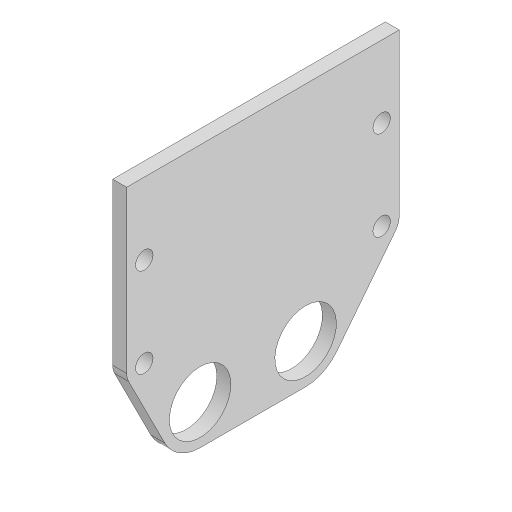
# Autodesk Inventor part: grabberPlate
Saved by Autodesk Inventor 2023 (Build 270158000, 158)
## iProperties
Created: 2022-09-10
Part Number: grabberPlate
Material: Generic
Document SubType Name: Modeling
Designer: deli
Density: 1 g/cm^3
Appearance: Default
Author: deli
Autodesk Inventor part; units mm, degrees
ref_plane "YZ Plane" through (0, 0, 0) normal (1, 0, 0) x (0, 1, 0)
ref_plane "XZ Plane" through (0, 0, 0) normal (0, 1, 0) x (-1, 0, 0)
ref_plane "XY Plane" through (0, 0, 0) normal (0, 0, 1) x (1, 0, 0)
sketch "Sketch1" plane through (0, 0, 0) normal (1, 0, 0) x (0, 1, 0)
  circle A0 centre (-43.9709, 92.2142) radius 2
  circle A1 centre (-43.9709, 38.2142) radius 2
  circle A2 centre (-57.9709, 55.5142) radius 4.99 construction
  circle A3 centre (-57.9709, 55.5142) radius 7
  circle A4 centre (-57.9709, 79.5142) radius 7
  line L0 (-57.9709, 79.5142) -> (-57.9709, 55.5142) construction
  line L1 (-45.779, 95.7822) -> (-62.0392, 87.5423)
  line L2 (-63.5162, 48.4255) -> (-46.4355, 35.0637)
  arc A5 (-43.9709, 96.2142) -> (-45.779, 95.7822) centre (-43.9709, 92.2142) ccw
  arc A6 (-46.4355, 35.0637) -> (-43.9709, 34.2142) centre (-43.9709, 38.2142) ccw
  line L3 (-43.9709, 96.2142) -> (-7.2969, 96.2142)
  line L4 (-7.2969, 34.2142) -> (-43.9709, 34.2142)
  arc A7 (-62.0392, 87.5423) -> (-66.9709, 79.5142) centre (-57.9709, 79.5142) ccw
  arc A8 (-66.9709, 55.5142) -> (-63.5162, 48.4255) centre (-57.9709, 55.5142) ccw
  line L5 (-66.9709, 55.5142) -> (-66.9709, 79.5142)
  line L6 (-43.9709, 38.2142) -> (-71.9709, 38.2142) construction
  line L7 (-71.9709, 92.2142) -> (-43.9709, 92.2142) construction
  line L8 (-7.2969, 96.2142) -> (-7.2969, 34.2142)
  circle A9 centre (-23.6339, 92.2142) radius 2
  circle A10 centre (-23.6339, 38.2142) radius 2
  point P0 (0, 0)
  dimension "d40" = 14
  dimension "d41" = 14
  dimension "d42" = 24
  dimension "d111" = 2
  dimension "d112" = 2
  dimension "d193" = 4
  dimension "d198" = 4
  dimension "d201" = 28
  dimension "d204" = 54
  dimension "d223" = 4
  dimension "d224" = 34.674
  dimension "d225" = 4
  dimension "d226" = 4
  dimension "d227" = 16.337
  dimension "d228" = 16.337
  constraints: 18 end point, 11 centre point, 8 point on circle, 5 tangent, 3 equal radius, 2 horizontal, 2 vertical, 1 coincident, 1 concentric, 3 other
  measures "d40" diameter of A3
  measures "d41" diameter of A4
  measures "d42" distance of L0.start L0.end
  measures "d111" radial gap between concentric circles of A4 A7
  measures "d112" radial gap between concentric circles of A3 A8
  measures "d193" diameter of A0
  measures "d198" diameter of A1
  measures "d201" distance of L7.start A0.centre
  measures "d204" distance of A1.centre A0.centre
  measures "d223" radius of A6
  measures "d224" distance edge to line of A0 L8
  measures "d225" distance from line of L3 A9.centre
  measures "d226" distance from line of L4 A10.centre
  measures "d227" distance from line of L8 A9.centre
  measures "d228" distance from line of L8 A10.centre
extrude "Extrusion2" add sketch "Sketch1" along normal blind 3.175
body "Solid2"
